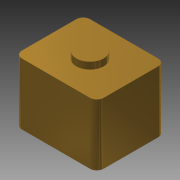
# Autodesk Inventor part: reducteur
Saved by Autodesk Inventor 2014 SP2 (Build 180246200, 246)
## iProperties
Created: 2015-03-17
Part Number: reducteur
Material: Laiton, jaune doux
Document SubType Name: Modeling
Designer: sd
Density: 8.47 g/cm^3
Appearance: Laiton - Satiné
Mass: 9.1886 g
Surface Area: 6.31398 cm^2
Volume: 1.08484 cm^3
Author: sd
Autodesk Inventor part; units mm, degrees
ref_plane "YZ Plane" through (0, 0, 0) normal (1, 0, 0) x (0, 1, 0)
ref_plane "XZ Plane" through (0, 0, 0) normal (0, 1, 0) x (-1, 0, 0)
ref_plane "XY Plane" through (0, 0, 0) normal (0, 0, 1) x (1, 0, 0)
sketch "Esquisse1" plane through (0, 0, 0) normal (0, 0, 1) x (1, 0, 0)
  line L0 (-6, -5) -> (6, -5)
  line L1 (6, -5) -> (6, 5)
  line L2 (6, 5) -> (-6, 5)
  line L3 (-6, 5) -> (-6, -5)
  point P0 (0, 0)
  dimension "d0" = 10
  dimension "d1" = 12
  dimension "d2" = 6
  dimension "d3" = 5
  constraints: 8 end point, 2 parallel, 1 horizontal, 1 perpendicular
  measures "d0" distance between parallel lines of L0 L2
  measures "d1" distance of L1.end L2.end
  measures "d2" horizontal distance of L2.end point (0, 0)
  measures "d3" vertical distance of point (0, 0) L0.end
extrude "Extrusion1" add sketch "Esquisse1" along normal blind 9
sketch "Esquisse2" plane through (0, 0, 9) normal (0, 0, 1) x (1, 0, 0)
  circle A0 centre (0, 0) radius 2
  dimension "d6" = 4
  constraints: 1 centre point, 1 coincident
  measures "d6" diameter of A0
extrude "Extrusion2" add sketch "Esquisse2" along normal blind 1
fillet "Congé1" radius 1 4 edges at (-6, 5, 4.5) (6, 5, 4.5) (6, -5, 4.5) (-6, -5, 4.5)
equation "\"d2\" = 0.5 * d1"
equation "\"d3\" = 0.5 * d0"
